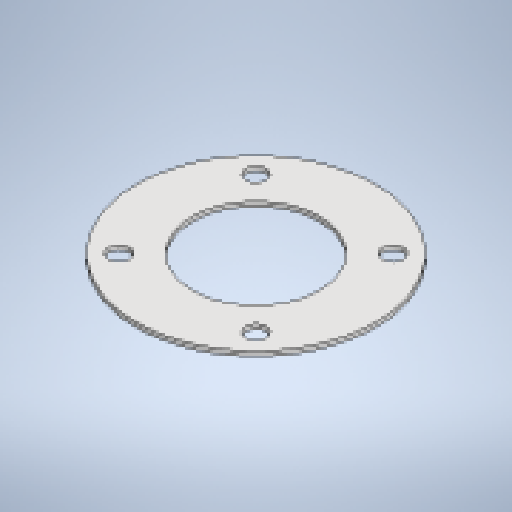
# Autodesk Inventor part: drain flange
Saved by Autodesk Inventor 2025 (Build 290162010, 162A)
## iProperties
Created: 2024-12-09
Part Number: drain flange
Material: Stainless Steel
Document SubType Name: Sheet Metal
Designer: user
Mass: 1674.72 g
Surface Area: 927.524 cm^2
Volume: 209.34 cm^3
Density: 8 g/cm^3
Sheet Metal Rule: AISI304 4mm Die 32
Sheet Metal Width: 210.000 mm
Sheet Metal Length: 210.000 mm
Sheet Metal Area: 44100.000 mm^2
Appearance: Default
Flat Pattern Width: 21 cm
Flat Pattern Length: 21 cm
Flat Pattern Area: 441 cm^2
Flange_D_outer: 210,000 mm
Flange_D1_hole_center: 170,000 mm
Flange_d_hole_diam: 18,000 mm
Flange_Tube_diam: 112.000 mm
Flange_number_of_hole: 4,000 ul
Author: user
Autodesk Inventor part; units mm, degrees
ref_plane "YZ Plane" through (0, 0, 0) normal (1, 0, 0) x (0, 1, 0)
ref_plane "XZ Plane" through (0, 0, 0) normal (0, 1, 0) x (-1, 0, 0)
ref_plane "XY Plane" through (0, 0, 0) normal (0, 0, 1) x (1, 0, 0)
sketch "Sketch1" plane through (0, 0, 0) normal (0, 0, 1) x (1, 0, 0)
  circle A0 centre (0, 0) radius 56
  circle A1 centre (0, 0) radius 105
  dimension "d22" = 112
  dimension "d23" = 210
  measures "d22" diameter of A0
  measures "d23" diameter of A1
extrude "Plate1" add sketch "Sketch1" along normal blind 4
sketch "Sketch5" plane through (0, 0, 4) normal (0, 0, 1) x (1, 0, 0)
  circle A0 centre (60.1041, 60.1041) radius 9
  circle A1 centre (0, 0) radius 85 construction
  line L0 (60.1041, 60.1041) -> (0, 0) construction
  line L1 (0, 0) -> (0, 85) construction
  dimension "d24" = 18
  dimension "d25" = 170
  dimension "d31" = 45
  constraints: 4 end point, 2 centre point, 2 point on circle, 1 coincident, 1 vertical
  measures "d24" diameter of A0
  measures "d25" diameter of A1
  measures "d31" angle of L1 L0
extrude "Cut1" cut sketch "Sketch5" against normal blind 4
pattern_circular "Circular Pattern1" count 4 over 360 about axis through (0, 0, 0) along (0, 0, 1) of "Cut1"
equation "\"d22\" = Flange_Tube_diam"
equation "\"d23\" = Flange_D_outer"
equation "\"d24\" = Flange_d_hole_diam"
equation "\"d25\" = Flange_D1_hole_center"
equation "\"d26\" = Thickness"
equation "\"d2\" = Thickness"
equation "\"BendReliefWidth\" = Thickness"
equation "\"BendReliefDepth\" = 0.5 * Thickness"
equation "\"CornerReliefSize\" = 4 * Thickness"
equation "\"MinimumRemnant\" = 2 * Thickness"
equation "\"TransitionRadius\" = BendRadius"
equation "\"JacobiRadiusSize\" = BendRadius"
equation "\"GapSize\" = Thickness"
equation "\"Flange_D_outer\" = 210"
equation "\"Flange_D1_hole_center\" = 170"
equation "\"Flange_d_hole_diam\" = 18"
equation "\"Flange_Tube_diam\" = 112"
equation "\"Thickness\" = 4"
equation "\"BendRadius\" = 6"
body "Solid1"
